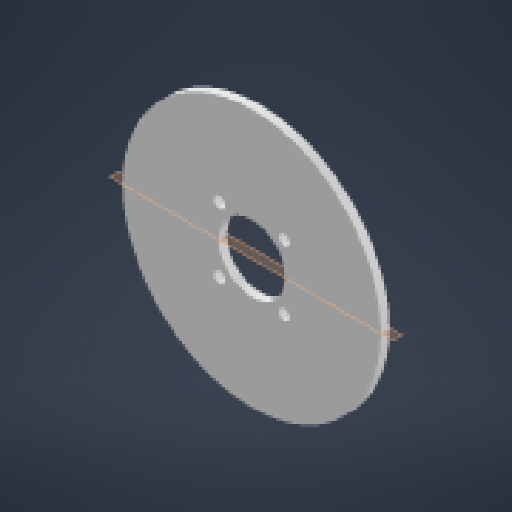
# Autodesk Inventor part: Flasque
Saved by Autodesk Inventor 2026.2 (Build 302298010, 298A)
## iProperties
Created: 2026-04-11
Part Number: Flasque
Material: Générique
Document SubType Name: Modeling
Designer: romai
Density: 1 g/cm^3
Appearance: Par défaut
Author: romai
Autodesk Inventor part; units mm, degrees
ref_plane "YZ Plane" through (0, 0, 0) normal (1, 0, 0) x (0, 1, 0)
ref_plane "XY Plane" through (0, 0, 0) normal (0, 0, 1) x (1, 0, 0)
sketch "Esquisse1" plane through (0, 0, 0) normal (0, 0, 1) x (1, 0, 0)
  circle A0 centre (0, 0) radius 77.5
  circle A1 centre (0, 0) radius 20
  dimension "d0" = 155
  dimension "d1" = 40
  constraints: 2 centre point, 2 coincident
  measures "d0" diameter of A0
  measures "d1" diameter of A1
extrude "Extrusion1" add sketch "Esquisse1" against normal blind 5
sketch "Esquisse2" plane through (0, 0, 0) normal (0, 0, 1) x (1, 0, 0)
  circle A0 centre (0, 0) radius 27.5
  line L0 (0, 0) -> (35.9549, 35.9549)
  line L1 (-108.5, 0) -> (108.5, 0) projected
  point P0 (19.4454, 19.4454)
  dimension "d11" = 55
  dimension "d15" = 45
  constraints: 2 end point, 1 coincident, 1 point on line, 3 other
  measures "d15" angle of L1 L0
hole "Perçage1" at (19.4454, 19.4454, 0) direction (0, 0, -1) diameter 6.6 end through all
pattern_circular "Réseau circulaire1" count 4 over 360 about axis through (0, 0, 0) along (0, 0, -1) of "Perçage1"
